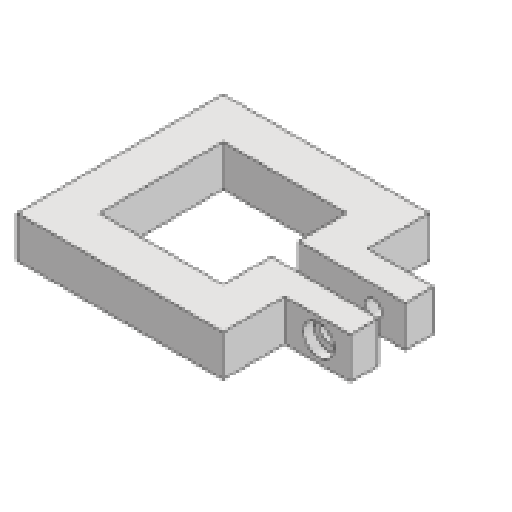
# Autodesk Inventor part: estopMountV2
Saved by Autodesk Inventor 2025 (Build 290162000, 162)
## iProperties
Created: 2024-11-24
Part Number: estopMountV2
Material: Generic
Document SubType Name: Modeling
Designer: derm
Density: 1 g/cm^3
Appearance: Default
Author: derm
Autodesk Inventor part; units mm, degrees
ref_plane "YZ Plane" through (0, 0, 0) normal (1, 0, 0) x (0, 1, 0)
ref_plane "XZ Plane" through (0, 0, 0) normal (0, 1, 0) x (-1, 0, 0)
ref_plane "XY Plane" through (0, 0, 0) normal (0, 0, 1) x (1, 0, 0)
sketch "Sketch1" plane through (0, 0, 0) normal (0, 1, 0) x (-1, 0, 0)
  line L0 (-15, 15) -> (15, 15)
  line L1 (15, 15) -> (15, -15)
  line L2 (15, -15) -> (-15, -15)
  line L3 (-15, 15) -> (15, -15) construction
  line L4 (15, 15) -> (-15, -15) construction
  line L5 (25, 25) -> (-25, 25)
  line L6 (-25.5008, -25) -> (24.4992, -25)
  line L7 (25, 25) -> (59.45, 25)
  line L8 (59.45, 25) -> (59.45, -25)
  line L9 (59.45, -25) -> (24.4992, -25)
  line L10 (-37.5196, -10.0467) -> (-25.5008, -10.0467)
  line L11 (-25, 10.0467) -> (-37.5196, 10.0467)
  line L12 (-37.5196, -3.2939) -> (-15, -3.2939)
  line L13 (-15, 3.2939) -> (-37.5196, 3.2939)
  line L14 (-37.5196, 10.0467) -> (-37.5196, 3.2939)
  line L15 (-37.5196, -3.2939) -> (-37.5196, -10.0467)
  line L16 (-25, 25) -> (-25, 10.0467)
  line L17 (-15, -15) -> (-15, -3.2939)
  line L18 (-15, 3.2939) -> (-15, 15)
  line L19 (-25.5008, -10.0467) -> (-25.5008, -25)
  point P0 (0, 0)
  point P1 (-30.7833, 0)
  point P2 (25, -25)
  dimension "d0" = 30
  dimension "d1" = 30
  dimension "d2" = 10
  dimension "d4" = 44.45
  constraints: 40 end point, 9 parallel, 4 horizontal, 2 midpoint, 2 perpendicular
  measures "d0" distance of L2.end L0.start
  measures "d1" distance of L1.end L2.end
  measures "d2" distance between parallel lines of L0 L5
  measures "d4" distance between parallel lines of L8 L1
extrude "Extrusion1" add sketch "Sketch1" along normal blind 10
sketch "Sketch2" plane through (0, 0, 0) normal (0, -1, 0) x (1, 0, 0)
  line L0 (15, 15) -> (-15, 15) projected
  line L1 (15, 3.2939) -> (15, 15) projected
  line L2 (37.5196, 3.2939) -> (15, 3.2939) projected
  line L3 (37.5196, 10.0467) -> (37.5196, 3.2939) projected
  line L4 (25, 10.0467) -> (37.5196, 10.0467) projected
  line L5 (25, 25) -> (25, 10.0467) projected
  line L6 (-59.45, 25) -> (25, 25) projected
  line L7 (-59.45, -25) -> (-59.45, 25) projected
  line L8 (25.5008, -25) -> (-59.45, -25) projected
  line L9 (25.5008, -10.0467) -> (25.5008, -25) projected
  line L10 (37.5196, -10.0467) -> (25.5008, -10.0467) projected
  line L11 (37.5196, -3.2939) -> (37.5196, -10.0467) projected
  line L12 (15, -3.2939) -> (37.5196, -3.2939) projected
  line L13 (15, -15) -> (15, -3.2939) projected
  line L14 (-15, -15) -> (15, -15) projected
  line L15 (-15, 15) -> (-15, -15) projected
  line L16 (-49.725, -25) -> (-24.725, -25)
  line L17 (-24.725, -25) -> (-24.725, 25)
  line L18 (-24.725, 25) -> (-49.725, 25)
  line L19 (-49.725, 25) -> (-49.725, -25)
  line L20 (-49.725, -25) -> (-24.725, 25) construction
  line L21 (-24.725, -25) -> (-49.725, 25) construction
  line L22 (-59.45, 25) -> (25, 25) projected
  line L23 (-15, 25) -> (-15, -25)
  line L24 (25.5008, -25) -> (-59.45, -25) projected
  line L25 (-59.45, 25) -> (-49.725, 25)
  line L26 (-59.45, 25) -> (25, 25) projected
  line L27 (-24.725, 25) -> (-15, 25)
  line L28 (-59.45, 21.5922) -> (-49.725, 21.5922)
  line L29 (-24.725, 21.5922) -> (-15, 21.5922)
  line L30 (-15, 15) -> (-15, -15) projected
  point P0 (0, 0)
  point P1 (-37.225, 0)
  point P2 (-15, -25)
  dimension "d7" = 25
  constraints: 22 end point, 9 point on line, 4 collinear, 3 perpendicular, 2 midpoint, 2 parallel, 1 horizontal
  measures "d7" distance between parallel lines of L19 L17
extrude "Extrusion2" add sketch "Sketch2" along normal blind 25 contours L15 L23 L8 L17 L29 | L29 L17 L6 L23 | L8 L7 L28 L19 | L19 L28 L7 L6
sketch "Sketch3" plane through (-24.725, 0, -25) normal (-1, 0, 0) x (0, 0, 1)
  line L0 (0, 0) -> (50, 0) construction
  line L1 (0, 0) -> (0, -25) construction
  line L2 (50, -25) -> (0, -25) construction
  line L3 (50, 0) -> (50, -25) construction
  line L4 (0, -12.5) -> (50, -12.5) construction
  line L5 (50, 0) -> (50, -25) construction
  line L6 (15, -12.5) -> (35, -12.5) construction
  line L7 (15, -15.2) -> (35, -15.2) construction
  line L8 (35, -9.8) -> (15, -9.8) construction
  arc A0 (15, -9.8) -> (15, -15.2) centre (15, -12.5) ccw construction
  arc A1 (35, -15.2) -> (35, -9.8) centre (35, -12.5) ccw
  circle A2 centre (35, -12.5) radius 2.7
  circle A3 centre (15, -12.5) radius 2.7
  point P0 (25, 0)
  point P1 (25, -12.5)
  point P2 (35, -9.8)
  dimension "d10" = 20
  dimension "d11" = 2.7
  constraints: 10 end point, 4 centre point, 4 midpoint, 4 point on circle, 4 tangent, 2 coincident, 1 concentric, 1 parallel, 1 point on line
  measures "d10" distance of L6.start L6.end
  measures "d11" radius of A0
extrude "Extrusion3" cut sketch "Sketch3" along normal through all both and the other way through all
sketch "Sketch4" plane through (37.5196, 0, 10.0467) normal (0, 0, 1) x (1, 0, 0)
  line L0 (-12.5196, 0) -> (0, 0) projected
  line L1 (0, 0) -> (0, 10) projected
  line L2 (-12.5196, 10) -> (0, 10) projected
  circle A0 centre (-5.6081, 5) radius 2
  line L3 (-12.5196, 0) -> (-12.5196, 10) projected
  point P0 (-37.5196, 0)
  dimension "d15" = 4
  constraints: 1 centre point
  measures "d15" diameter of A0
extrude "Extrusion4" cut sketch "Sketch4" against normal through all contours A0
sketch "Sketch5" plane through (37.5196, 0, 10.0467) normal (0, 0, 1) x (1, 0, 0)
  circle A0 centre (-5.6081, 5) radius 2 projected
  circle A1 centre (-5.6081, 5) radius 3.6921
  point P0 (-37.5196, 0)
  point P1 (-9.307, 3.7757)
  point P2 (-9.307, 6.2243)
  constraints: 1 centre point, 1 coincident, 1 other
extrude "Extrusion5" cut sketch "Sketch5" along normal mid plane 5 contours A0 | A1
sketch "Sketch6" plane through (0, 10, 0) normal (0, 1, 0) x (1, 0, 0)
  line L0 (25, -25) -> (25, -10.0467) projected
  line L1 (25, -10.0467) -> (37.5196, -10.0467) projected
  line L2 (37.5196, -10.0467) -> (37.5196, -3.2939) projected
  line L3 (37.5196, -3.2939) -> (15, -3.2939) projected
  line L4 (15, -3.2939) -> (15, -15) projected
  line L5 (15, -15) -> (-15, -15) projected
  line L6 (-15, -15) -> (-15, 15) projected
  line L7 (-15, 15) -> (15, 15) projected
  line L8 (15, 15) -> (15, 3.2939) projected
  line L9 (15, 3.2939) -> (37.5196, 3.2939) projected
  line L10 (37.5196, 3.2939) -> (37.5196, 10.0467) projected
  line L11 (37.5196, 10.0467) -> (25.5008, 10.0467) projected
  line L12 (25.5008, 10.0467) -> (25.5008, 25) projected
  line L13 (25.5008, 25) -> (-59.45, 25) projected
  line L14 (-59.45, 25) -> (-59.45, -25) projected
  line L15 (-59.45, -25) -> (25, -25) projected
  line L16 (-59.45, -25) -> (20, -25) projected
  line L17 (-25, -25) -> (-25, 25)
  point P0 (0, 0)
  dimension "d20" = 10
  dimension "d21" = 10
  constraints: 2 end point, 2 point on line, 1 perpendicular
  measures "d20" distance between parallel lines of L6 L17
  measures "d21" distance between parallel lines of L15 L5
extrude "Extrusion6" cut sketch "Sketch6" against normal through all contours L15 L14 L13 L17
sketch "Sketch7" plane through (-24.725, 0, -25) normal (-1, 0, 0) x (0, 0, 1)
  circle A0 centre (35, -12.5) radius 2.7 projected
  circle A1 centre (15, -12.5) radius 2.7 projected
  line L0 (50, -25) -> (0, -25) projected
  line L1 (50, 0) -> (50, -25) projected
  line L2 (0, 0) -> (50, 0) projected
  line L3 (0, 0) -> (0, -25) projected
  point P0 (25, 0)
extrude "Extrusion7" cut sketch "Sketch7" against normal through all
sketch "Sketch8" plane through (-25, 10, -25) normal (-1, 0, 0) x (0, 0, 1)
  line L0 (50, -10) -> (0, -10) projected
  line L1 (50, 0) -> (50, -10) projected
  line L2 (0, 0) -> (50, 0) projected
  line L3 (0, -10) -> (0, 0) projected
  point P0 (25, -10)
extrude "Extrusion8" add sketch "Sketch8" along normal blind 15
sketch "Sketch9" plane through (37.5196, 0, -10.0467) normal (0, 0, -1) x (-1, 0, 0)
  circle A0 centre (5.6081, 5) radius 2 projected
  line L0 (0, 0) -> (12.0187, 0) projected
  line L1 (12.0187, 0) -> (12.0187, 10) projected
  line L2 (0, 10) -> (12.0187, 10) projected
  line L3 (0, 0) -> (0, 10) projected
  circle A1 centre (5.6081, 5) radius 3.6921 projected
  line L4 (7.9753, 9.1) -> (10.3424, 5)
  line L5 (10.3424, 5) -> (7.9753, 0.9)
  line L6 (7.9753, 0.9) -> (3.241, 0.9)
  line L7 (3.241, 0.9) -> (0.8739, 5)
  line L8 (0.8739, 5) -> (3.241, 9.1)
  line L9 (3.241, 9.1) -> (7.9753, 9.1)
  point P0 (37.5196, 0)
  point P1 (8.8062, 2.3392)
  point P2 (8.8062, 7.6608)
  point P3 (8.8062, 6.8449)
  point P4 (8.8062, 3.1551)
  dimension "d28" = 8.2
  constraints: 12 end point, 1 coincident, 1 parallel, 13 other
  measures "d28" distance between parallel lines of L9 L6
extrude "Extrusion9" add sketch "Sketch9" along normal up to surface (14.9533 mm away) contours L3 L2 L1 L0
sketch "Sketch10" plane through (25, 0, 10.0467) normal (0, 0, 1) x (1, 0, 0)
  circle A0 centre (6.9114, 5) radius 3.6921 projected
  line L0 (0, 0) -> (12.5196, 0) projected
  line L1 (12.5196, 0) -> (12.5196, 10) projected
  line L2 (0, 10) -> (12.5196, 10) projected
  line L3 (0, 0) -> (0, 10) projected
  point P0 (-25, 0)
extrude "Extrusion10" add sketch "Sketch10" along normal up to surface (14.9533 mm away)
sketch "Sketch11" plane through (0, 10, 0) normal (0, 1, 0) x (1, 0, 0)
  line L0 (-40.28, -55.2921) -> (-40.28, 159.5519) projected
  line L1 (-15.12, -75.3901) -> (-15.12, 179.6099) projected
  line L2 (-40, -25) -> (37.5196, -25) projected
  line L3 (37.5196, -3.2939) -> (37.5196, -25) projected
  line L4 (37.5196, -3.2939) -> (15, -3.2939) projected
  line L5 (15, -3.2939) -> (15, -15) projected
  line L6 (15, -15) -> (-15, -15) projected
  line L7 (-15, -15) -> (-15, 15) projected
  line L8 (-15, 15) -> (15, 15) projected
  line L9 (15, 15) -> (15, 3.2939) projected
  line L10 (15, 3.2939) -> (37.5196, 3.2939) projected
  line L11 (37.5196, 3.2939) -> (37.5196, 25) projected
  line L12 (37.5196, 25) -> (-40, 25) projected
  line L13 (-40, -25) -> (-40, 25) projected
  line L14 (-15.12, 25) -> (-40, 25) construction
  circle A0 centre (-27.56, 15) radius 2.75
  circle A1 centre (-27.56, -15) radius 2.75
  point P0 (0, 0)
  dimension "d33" = 5.5
  constraints: 2 centre point, 2 end point, 2 point on line, 1 collinear, 1 equal radius
  measures "d33" diameter of A0
extrude "Extrusion11" cut sketch "Sketch11" against normal through all contours A0 | A1
fillet "Fillet2" radius 10 4 edges at (37.5196, 5, 25) (37.5196, 5, -25) (-40, 5, 25) (-40, 5, -25)
body "Solid1"
